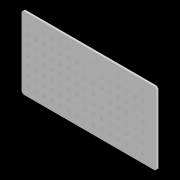
# Autodesk Inventor part: Part4
Saved by Autodesk Inventor 2020.4 (Build 244396010, 396A)
## iProperties
Created: 2022-09-20
Part Number: Part4
Material: Generic
Document SubType Name: Modeling
Designer: Val
Density: 1 g/cm^3
Appearance: Default
Author: Val
Autodesk Inventor part; units mm, degrees
ref_plane "YZ Plane" through (0, 0, 0) normal (1, 0, 0) x (0, 1, 0)
ref_plane "XZ Plane" through (0, 0, 0) normal (0, 1, 0) x (-1, 0, 0)
ref_plane "XY Plane" through (0, 0, 0) normal (0, 0, 1) x (1, 0, 0)
sketch "Sketch1" plane through (0, 0, 0) normal (0, 0, 1) x (1, 0, 0)
  line L0 (-533.7919, 263.0154) -> (507.6081, 263.0154)
  line L1 (507.6081, 263.0154) -> (507.6081, -295.7846)
  line L2 (507.6081, -295.7846) -> (-533.7919, -295.7846)
  line L3 (-533.7919, -295.7846) -> (-533.7919, 263.0154)
  point P0 (0, 0)
  dimension "d0" = 558.8
  dimension "d1" = 1041.4
  constraints: 8 end point, 2 parallel, 1 horizontal, 1 perpendicular
  measures "d0" distance of L2.end L0.start
  measures "d1" distance of L0.start L0.end
extrude "Extrusion1" add sketch "Sketch1" along normal blind 12.7
sketch "Sketch2" plane through (0, 0, 12.7) normal (0, 0, 1) x (1, 0, 0)
  line L0 (-533.7919, 263.0154) -> (-533.7919, -295.7846) construction
  line L1 (-533.7919, 193.1654) -> (507.6081, 193.1654) construction
  line L2 (507.6081, -295.7846) -> (507.6081, 263.0154) construction
  line L3 (-533.7919, 123.3154) -> (507.6081, 123.3154) construction
  line L4 (-533.7919, 53.4654) -> (507.6081, 53.4654) construction
  line L5 (-533.7919, -16.3846) -> (507.6081, -16.3846) construction
  line L6 (507.6081, 263.0154) -> (-533.7919, 263.0154) construction
  line L7 (-483.7919, 263.0154) -> (-483.7919, -16.3846) construction
  circle A0 centre (-483.7919, 193.1654) radius 5
  circle A1 centre (-483.7919, 123.3154) radius 5
  circle A2 centre (-483.7919, 53.4654) radius 5
  circle A3 centre (-483.7919, -16.3846) radius 5
  circle A4 centre (-483.7919, -225.9346) radius 5
  circle A5 centre (-483.7919, -156.0846) radius 5
  circle A6 centre (-483.7919, -86.2346) radius 5
  circle A7 centre (-483.7919, -16.3846) radius 5
  circle A8 centre (-420.2919, 193.1654) radius 5
  circle A9 centre (-420.2919, 123.3154) radius 5
  circle A10 centre (-420.2919, 53.4654) radius 5
  circle A11 centre (-420.2919, -16.3846) radius 5
  circle A12 centre (-420.2919, -86.2346) radius 5
  circle A13 centre (-420.2919, -156.0846) radius 5
  circle A14 centre (-420.2919, -225.9346) radius 5
  circle A15 centre (-356.7919, 193.1654) radius 5
  circle A16 centre (-356.7919, 123.3154) radius 5
  circle A17 centre (-356.7919, 53.4654) radius 5
  circle A18 centre (-356.7919, -16.3846) radius 5
  circle A19 centre (-356.7919, -86.2346) radius 5
  circle A20 centre (-356.7919, -156.0846) radius 5
  circle A21 centre (-356.7919, -225.9346) radius 5
  circle A22 centre (-293.2919, 193.1654) radius 5
  circle A23 centre (-293.2919, 123.3154) radius 5
  circle A24 centre (-293.2919, 53.4654) radius 5
  circle A25 centre (-293.2919, -16.3846) radius 5
  circle A26 centre (-293.2919, -86.2346) radius 5
  circle A27 centre (-293.2919, -156.0846) radius 5
  circle A28 centre (-293.2919, -225.9346) radius 5
  circle A29 centre (-229.7919, 193.1654) radius 5
  circle A30 centre (-229.7919, 123.3154) radius 5
  circle A31 centre (-229.7919, 53.4654) radius 5
  circle A32 centre (-229.7919, -16.3846) radius 5
  circle A33 centre (-229.7919, -86.2346) radius 5
  circle A34 centre (-229.7919, -156.0846) radius 5
  circle A35 centre (-229.7919, -225.9346) radius 5
  circle A36 centre (-166.2919, 193.1654) radius 5
  circle A37 centre (-166.2919, 123.3154) radius 5
  circle A38 centre (-166.2919, 53.4654) radius 5
  circle A39 centre (-166.2919, -16.3846) radius 5
  circle A40 centre (-166.2919, -86.2346) radius 5
  circle A41 centre (-166.2919, -156.0846) radius 5
  circle A42 centre (-166.2919, -225.9346) radius 5
  circle A43 centre (-102.7919, 193.1654) radius 5
  circle A44 centre (-102.7919, 123.3154) radius 5
  circle A45 centre (-102.7919, 53.4654) radius 5
  circle A46 centre (-102.7919, -16.3846) radius 5
  circle A47 centre (-102.7919, -86.2346) radius 5
  circle A48 centre (-102.7919, -156.0846) radius 5
  circle A49 centre (-102.7919, -225.9346) radius 5
  circle A50 centre (-39.2919, 193.1654) radius 5
  circle A51 centre (-39.2919, 123.3154) radius 5
  circle A52 centre (-39.2919, 53.4654) radius 5
  circle A53 centre (-39.2919, -16.3846) radius 5
  circle A54 centre (-39.2919, -86.2346) radius 5
  circle A55 centre (-39.2919, -156.0846) radius 5
  circle A56 centre (-39.2919, -225.9346) radius 5
  circle A57 centre (24.2081, 193.1654) radius 5
  circle A58 centre (24.2081, 123.3154) radius 5
  circle A59 centre (24.2081, 53.4654) radius 5
  circle A60 centre (24.2081, -16.3846) radius 5
  circle A61 centre (24.2081, -86.2346) radius 5
  circle A62 centre (24.2081, -156.0846) radius 5
  circle A63 centre (24.2081, -225.9346) radius 5
  circle A64 centre (87.7081, 193.1654) radius 5
  circle A65 centre (87.7081, 123.3154) radius 5
  circle A66 centre (87.7081, 53.4654) radius 5
  circle A67 centre (87.7081, -16.3846) radius 5
  circle A68 centre (87.7081, -86.2346) radius 5
  circle A69 centre (87.7081, -156.0846) radius 5
  circle A70 centre (87.7081, -225.9346) radius 5
  circle A71 centre (151.2081, 193.1654) radius 5
  circle A72 centre (151.2081, 123.3154) radius 5
  circle A73 centre (151.2081, 53.4654) radius 5
  circle A74 centre (151.2081, -16.3846) radius 5
  circle A75 centre (151.2081, -86.2346) radius 5
  circle A76 centre (151.2081, -156.0846) radius 5
  circle A77 centre (151.2081, -225.9346) radius 5
  circle A78 centre (214.7081, 193.1654) radius 5
  circle A79 centre (214.7081, 123.3154) radius 5
  circle A80 centre (214.7081, 53.4654) radius 5
  circle A81 centre (214.7081, -16.3846) radius 5
  circle A82 centre (214.7081, -86.2346) radius 5
  circle A83 centre (214.7081, -156.0846) radius 5
  circle A84 centre (214.7081, -225.9346) radius 5
  circle A85 centre (278.2081, 193.1654) radius 5
  circle A86 centre (278.2081, 123.3154) radius 5
  circle A87 centre (278.2081, 53.4654) radius 5
  circle A88 centre (278.2081, -16.3846) radius 5
  circle A89 centre (278.2081, -86.2346) radius 5
  circle A90 centre (278.2081, -156.0846) radius 5
  circle A91 centre (278.2081, -225.9346) radius 5
  circle A92 centre (341.7081, 193.1654) radius 5
  circle A93 centre (341.7081, 123.3154) radius 5
  circle A94 centre (341.7081, 53.4654) radius 5
  circle A95 centre (341.7081, -16.3846) radius 5
  circle A96 centre (341.7081, -86.2346) radius 5
  circle A97 centre (341.7081, -156.0846) radius 5
  circle A98 centre (341.7081, -225.9346) radius 5
  circle A99 centre (405.2081, 193.1654) radius 5
  circle A100 centre (405.2081, 123.3154) radius 5
  circle A101 centre (405.2081, 53.4654) radius 5
  circle A102 centre (405.2081, -16.3846) radius 5
  circle A103 centre (405.2081, -86.2346) radius 5
  circle A104 centre (405.2081, -156.0846) radius 5
  circle A105 centre (405.2081, -225.9346) radius 5
  point P0 (0, 0)
  dimension "d4" = 279.4
  dimension "d5" = 69.85
  dimension "d6" = 69.85
  dimension "d7" = 69.85
  dimension "d8" = 50
  dimension "d9" = 10
  dimension "d10" = 10
  dimension "d11" = 10
  dimension "d12" = 10
  dimension "d15" = 63.5
  constraints: 106 centre point, 12 point on line, 10 end point, 4 perpendicular, 3 midpoint, 3 symmetric about line, 2 horizontal, 1 coincident, 200 other
  measures "d4" distance between parallel lines of L5 L6
  measures "d5" distance between parallel lines of L5 L4
  measures "d6" distance between parallel lines of L3 L4
  measures "d7" distance between parallel lines of L1 L3
  measures "d8" distance between parallel lines of L0 L7
  measures "d9" diameter of A0
  measures "d10" diameter of A1
  measures "d11" diameter of A2
  measures "d12" diameter of A3
  measures "d15" distance of A0.centre A8.centre
extrude "Extrusion2" cut sketch "Sketch2" against normal through all
chamfer "Chamfer1" distance 12.7 angle 45 4 edges at (-533.7919, -295.7846, 6.35) (-533.7919, 263.0154, 6.35) (507.6081, 263.0154, 6.35) (507.6081, -295.7846, 6.35)
equation "\"d5\" = 0.25 * d4"
equation "\"d6\" = 0.25 * d4"
equation "\"d7\" = 0.25 * d4"
body "Solid1"
